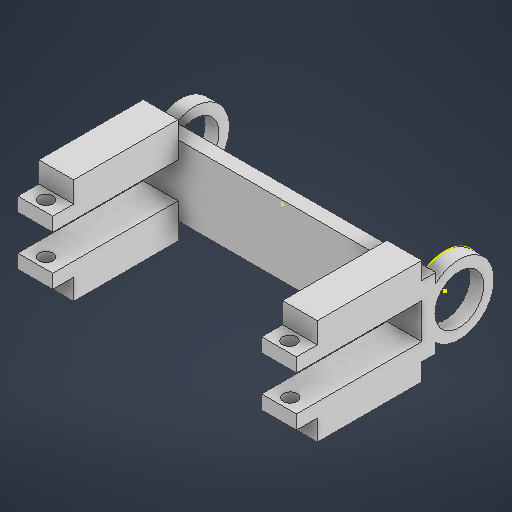
# Autodesk Inventor part: mount
Saved by Autodesk Inventor 2026.1 (Build 301233020, 233B)
## iProperties
Created: 2026-01-27
Part Number: mount
Material: Generic
Document SubType Name: Modeling
Designer: Dylan
Density: 1 g/cm^3
Appearance: Default
Author: Dylan
Autodesk Inventor part; units mm, degrees
ref_plane "YZ Plane" through (0, 0, 0) normal (1, 0, 0) x (0, 1, 0)
ref_plane "XZ Plane" through (0, 0, 0) normal (0, 1, 0) x (-1, 0, 0)
ref_plane "XY Plane" through (0, 0, 0) normal (0, 0, 1) x (1, 0, 0)
sketch "Sketch3" plane through (0, 0, 0) normal (0, 1, 0) x (-1, 0, 0)
  line L0 (-14.9997, 0) -> (-19.9997, 0)
  line L1 (-19.9997, 0) -> (-19.9997, 15)
  line L2 (-19.9997, 15) -> (-14.9997, 15)
  line L3 (-14.9997, 15) -> (-14.9997, 0)
  line L4 (14.9998, 0) -> (19.9998, 0)
  line L5 (19.9998, 0) -> (19.9998, 15)
  line L6 (19.9998, 15) -> (14.9998, 15)
  line L7 (14.9998, 15) -> (14.9998, 0)
  point P0 (0, 0)
  dimension "d4" = 5
  dimension "d5" = 15
  dimension "d6" = 5
  dimension "d7" = 15
  constraints: 16 end point, 4 parallel, 2 horizontal, 2 perpendicular
  measures "d4" distance of L1.end L2.end
  measures "d5" distance of L0.end L1.end
  measures "d6" distance of L6.end L5.end
  measures "d7" distance of L5.end L4.end
extrude "Extrusion1" add sketch "Sketch3" along normal blind 5
sketch "Sketch5" plane through (-19.9998, 0, 15) normal (0, 0, 1) x (1, 0, 0)
  line L0 (5, 0) -> (0, 0) projected
  line L1 (0, 0) -> (5, 0)
  line L2 (5, 0) -> (5, 2)
  line L3 (5, 2) -> (0, 2)
  line L4 (0, 2) -> (0, 0)
  line L5 (34.9995, 0) -> (39.9995, 0) projected
  line L6 (34.9995, 0) -> (39.9995, 0)
  line L7 (39.9995, 0) -> (39.9995, 2)
  line L8 (39.9995, 2) -> (34.9995, 2)
  line L9 (34.9995, 2) -> (34.9995, 0)
  point P0 (19.9998, 0)
  dimension "d10" = 5
  dimension "d11" = 2
  dimension "d12" = 5
  dimension "d13" = 2
  constraints: 16 end point, 4 parallel, 2 horizontal, 2 perpendicular
  measures "d10" distance of L3.end L2.end
  measures "d11" distance of L2.end L1.end
  measures "d12" distance of L8.end L7.end
  measures "d13" distance of L7.end L6.end
extrude "Extrusion2" add sketch "Sketch5" along normal blind 3
sketch "Sketch6" plane through (-19.9998, 2, 15) normal (0, 1, 0) x (1, 0, 0)
  point P0 (19.9998, 15)
sketch "Sketch7" plane through (-19.9998, 2, 15) normal (0, 1, 0) x (1, 0, 0)
  circle A0 centre (2.5, -1.466) radius 1
  line L0 (0, 0) -> (0, -3) projected
  circle A1 centre (37.4995, -1.5) radius 1
  line L1 (34.9995, 0) -> (34.9995, -3) projected
  point P0 (19.9998, 15)
  point P1 (0, -1.5)
  point P2 (34.9995, -1.5)
  dimension "d16" = 2
  dimension "d17" = 2.5
  dimension "d18" = 2
  dimension "d19" = 2.5
  constraints: 2 centre point, 2 midpoint
  measures "d16" diameter of A0
  measures "d17" horizontal distance of point (0, -1.5) A0.centre
  measures "d18" diameter of A1
  measures "d19" distance of point (35, -1.5) A1.centre
extrude "Extrusion3" cut sketch "Sketch7" against normal blind 2
sketch "Sketch8" plane through (19.9997, 0, 0) normal (0, 0, -1) x (-1, 0, 0)
  line L0 (0, 2) -> (0, 5) projected
  line L1 (0, 2.5002) -> (40, 2.5002)
  line L2 (40, 2.5002) -> (40, -7.5998)
  line L3 (40, -7.5998) -> (0, -7.5998)
  line L4 (0, -7.5998) -> (0, 2.5002)
  point P0 (19.9997, 0)
  dimension "d22" = 40
  dimension "d23" = 10.1
  constraints: 8 end point, 2 parallel, 1 horizontal, 1 perpendicular, 1 point on line
  measures "d22" distance of L2.end L3.end
  measures "d23" distance of L1.end L2.end
extrude "Extrusion4" add sketch "Sketch8" along normal blind 2
sketch "Sketch9" plane through (19.9997, 0, 0) normal (0, 0, 1) x (1, 0, 0)
  line L0 (-40, -7.5998) -> (-40, 2.5002) projected
  line L1 (-40, -5.1) -> (-35, -5.1)
  line L2 (-35, -5.1) -> (-35, -10.1)
  line L3 (-35, -10.1) -> (-40, -10.1)
  line L4 (-40, -10.1) -> (-40, -5.1)
  line L5 (0, 0) -> (0, -7.5998) projected
  line L6 (0, -5.1) -> (-5, -5.1)
  line L7 (-5, -5.1) -> (-5, -10.1)
  line L8 (-5, -10.1) -> (0, -10.1)
  line L9 (0, -10.1) -> (0, -5.1)
  point P0 (-19.9997, 0)
  dimension "d26" = 5
  dimension "d27" = 5
  dimension "d28" = 5
  dimension "d29" = 5
  constraints: 16 end point, 4 parallel, 3 point on line, 2 horizontal, 2 perpendicular
  measures "d26" distance of L2.end L3.end
  measures "d27" distance of L1.end L2.end
  measures "d28" distance of L8.end L7.end
  measures "d29" distance of L7.end L6.end
extrude "Extrusion5" add sketch "Sketch9" along normal blind 15
sketch "Sketch10" plane through (19.9997, 0, 15) normal (0, 0, 1) x (1, 0, 0)
  line L0 (-35, -5.1) -> (-40, -5.1)
  line L1 (-40, -5.1) -> (-40, -7.1)
  line L2 (-40, -7.1) -> (-35, -7.1)
  line L3 (-35, -7.1) -> (-35, -5.1)
  line L4 (-5, -5.1) -> (-5, -10.1) projected
  line L5 (-5, -5.1) -> (0, -5.1)
  line L6 (0, -5.1) -> (0, -7.1)
  line L7 (0, -7.1) -> (-5, -7.1)
  line L8 (-5, -7.1) -> (-5, -5.1)
  point P0 (-19.9997, 0)
  dimension "d32" = 5
  dimension "d33" = 2
  dimension "d34" = 5
  dimension "d35" = 2
  constraints: 16 end point, 4 parallel, 2 horizontal, 2 perpendicular
  measures "d32" distance of L2.end L1.end
  measures "d33" distance of L1.end L0.end
  measures "d34" distance of L6.end L7.end
  measures "d35" distance of L5.end L6.end
extrude "Extrusion6" add sketch "Sketch10" along normal blind 3
sketch "Sketch11" plane through (-20.0003, -7.1, 15) normal (0, -1, 0) x (1, 0, 0)
  circle A0 centre (2.4996, 1.4564) radius 1
  line L0 (0, 0) -> (0, 3) projected
  circle A1 centre (37.5, 1.4063) radius 1
  line L1 (40, 0) -> (40, 3) projected
  point P0 (20.0003, -15)
  point P1 (0, 1.5)
  point P2 (40, 1.5)
  dimension "d38" = 2
  dimension "d39" = 2.5
  dimension "d40" = 2
  dimension "d41" = 2.5
  constraints: 2 centre point, 2 midpoint
  measures "d38" diameter of A0
  measures "d39" distance of point (0, 1.5) A0.centre
  measures "d40" diameter of A1
  measures "d41" horizontal distance of point (40, 1.5) A1.centre
extrude "Extrusion7" cut sketch "Sketch11" against normal blind 2
sketch "Sketch13" plane through (19.9997, 5, 15) normal (1, 0, 0) x (0, 0, -1)
  circle A0 centre (20.3727, -7.5498) radius 5
  point P0 (15, -5)
  dimension "d44" = 10
  constraints: 1 centre point
  measures "d44" diameter of A0
extrude "Extrusion8" add sketch "Sketch13" against normal blind 2
sketch "Sketch14" plane through (17.9997, 5, 15) normal (-1, 0, 0) x (0, 0, 1)
  arc A0 (-17, -3.8586) -> (-17, -11.241) centre (-20.3727, -7.5498) ccw projected
  point P0 (-15, -5)
sketch "Sketch15" plane through (-20.0003, -7.5998, -2) normal (-1, 0, 0) x (0, 0, 1)
  point P0 (2, 7.5998)
sketch "Sketch16" plane through (-20.0003, -7.5998, -2) normal (-1, 0, 0) x (0, 0, 1)
  circle A0 centre (-3.3725, 5.0498) radius 5
  point P0 (2, 7.5998)
  dimension "d47" = 10
  constraints: 1 centre point
  measures "d47" diameter of A0
extrude "Extrusion9" add sketch "Sketch16" against normal blind 2
sketch "Sketch18" plane through (-20.0003, 2.5002, -2) normal (-1, 0, 0) x (0, 0, 1)
  arc A0 (0, -1.3588) -> (0, -8.7412) centre (-3.3727, -5.05) ccw projected
  circle A1 centre (-3.3727, -5.05) radius 3.5
  point P0 (2, -2.5002)
  dimension "d50" = 7
  constraints: 1 centre point, 1 coincident
  measures "d50" diameter of A1
extrude "Extrusion10" cut sketch "Sketch18" against normal blind 40
body "Solid1"
